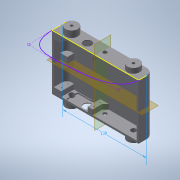
# Autodesk Inventor part: base-v2
Saved by Autodesk Inventor 2020 (Build 240168000, 168)
## iProperties
Created: 2020-08-23
Part Number: base-v2
Material: Ogólny
Document SubType Name: Modeling
Designer: blep
Density: 1 g/cm^3
Appearance: Domyślna
Author: blep
Autodesk Inventor part; units mm, degrees
ref_plane "YZ Plane" through (0, 0, 0) normal (1, 0, 0) x (0, 1, 0)
ref_plane "XZ Plane" through (0, 0, 0) normal (0, 1, 0) x (-1, 0, 0)
ref_plane "XY Plane" through (0, 0, 0) normal (0, 0, 1) x (1, 0, 0)
sketch "Szkic1" plane through (0, 0, 0) normal (0, 0, 1) x (1, 0, 0)
  line L0 (0, 0) -> (135, 0)
  line L1 (135, 0) -> (135, -86)
  line L2 (135, -86) -> (0, -86)
  line L3 (0, -86) -> (0, 0)
  line L4 (3, -3) -> (132, -3)
  line L5 (132, -3) -> (132, -83)
  line L6 (132, -83) -> (3, -83)
  line L7 (3, -83) -> (3, -3)
  dimension "d0" = 86
  dimension "d1" = 135
  dimension "d2" = 3
  constraints: 16 end point, 4 parallel, 2 perpendicular, 1 horizontal, 3 other
  measures "d0" distance of L0.end L1.end
  measures "d1" distance of L1.end L2.end
  measures "d2" distance between parallel lines of L3 L7
extrude "Wyciągnięcie proste1" add sketch "Szkic1" against normal blind 3 contours L0 L1 L2 L3 | L4 L5 L6 L7
extrude "Wyciągnięcie proste2" add sketch "Szkic1" along normal blind 20
sketch "Szkic2" plane through (0, 0, -3) normal (0, 1, 0) x (1, 0, 0)
  line L0 (135, 0) -> (135, -23) projected
  line L1 (0, 0) -> (135, 0) projected
  line L2 (0, 0) -> (0, -23) projected
  line L3 (135, -23) -> (0, -23) projected
  line L4 (115.75, -11.5) -> (19.25, -11.5)
  line L5 (135, -23) -> (115.75, -11.5) construction
  line L6 (0, 0) -> (135, 0) construction
  line L7 (115.75, -11.5) -> (135, 0) construction
  line L8 (135, -23) -> (0, -23) construction
  line L9 (19.25, -11.5) -> (0, -23) construction
  point P0 (0, -3)
  dimension "d7" = 96.5
  constraints: 8 end point, 2 equal length, 1 horizontal
  measures "d7" distance of L4.start L4.end
hole "Otwór1" at (19.25, 0, 8.5) at (115.75, 0, 8.5) direction (0, -1, 0) diameter 4.25 end through all
sketch "Szkic3" plane through (0, 0, -3) normal (0, 1, 0) x (1, 0, 0)
  circle A0 centre (19.25, -11.5) radius 2.125 projected
  circle A1 centre (19.25, -11.5) radius 10 projected
  circle A2 centre (19.25, -11.5) radius 9.5
  circle A3 centre (115.75, -11.5) radius 2.125 projected
  circle A4 centre (115.75, -11.5) radius 2.125 projected
  circle A5 centre (115.75, -11.5) radius 9.5
  point P0 (0, -3)
  dimension "d15" = 0.5
  constraints: 2 centre point, 1 coincident, 1 equal radius
  measures "d15" radial gap between concentric circles of A1 A2
extrude "Wyciągnięcie proste3" add sketch "Szkic3" along normal blind 10 contours A2
extrude "Wyciągnięcie proste4" add sketch "Szkic3" along normal blind 7.6 contours A5
ref_plane "Płaszczyzna konstrukcyjna1" through (0, -43, -3) normal (0, 1, 0) x (1, 0, 0)
mirror "Odbij1" about plane through (0, -43, -3) normal (0, 1, 0) of "Wyciągnięcie proste3", "Wyciągnięcie proste4"
ref_plane "Płaszczyzna konstrukcyjna2" through (0, -43, -3) normal (0, 1, 0) x (1, 0, 0)
sketch "Szkic4" plane through (3, -83, 0) normal (0, 1, 0) x (1, 0, 0)
  circle A0 centre (16.25, -8.5) radius 2.125 projected
  circle A1 centre (112.75, -8.5) radius 2.125 projected
  circle A2 centre (112.75, -8.5) radius 4
  circle A3 centre (16.25, -8.5) radius 4
  point P0 (-3, 0)
  dimension "d20" = 8
  dimension "d21" = 8
  constraints: 2 centre point, 2 coincident
  measures "d20" diameter of A2
  measures "d21" diameter of A3
extrude "Wyciągnięcie proste5" cut sketch "Szkic4" against normal blind 10 contours A0 | A3
extrude "Wyciągnięcie proste6" cut sketch "Szkic4" against normal blind 7.6 contours A1 | A2
mirror "Odbij2" about plane through (0, -43, -3) normal (0, 1, 0) of "Wyciągnięcie proste5", "Wyciągnięcie proste6"
sketch "Szkic5" plane through (3, -83, 0) normal (0, 1, 0) x (1, 0, 0)
  arc A0 (12, -18.8) -> (12.7, -19.5) centre (12.7, -18.8) ccw projected
  line L0 (12, -18.8) -> (12, -1) projected
  arc A1 (12.7, -0.3) -> (12, -1) centre (12.7, -1) ccw projected
  line L1 (12.7, -0.3) -> (42.3, -0.3) projected
  arc A2 (42.3, -0.3) -> (38.7014, -1) centre (42.3, -9.9) ccw projected
  line L2 (38.7014, -1) -> (19.4014, -1) projected
  arc A3 (19.4014, -1) -> (18.4014, -2) centre (19.4014, -2) ccw projected
  line L3 (18.4014, -2) -> (18.4014, -4.6756) projected
  arc A4 (18.4014, -4.6756) -> (18.4014, -14.0756) centre (22.3218, -9.3756) ccw projected
  line L4 (18.4014, -14.0756) -> (18.4014, -17.8) projected
  arc A5 (18.4014, -17.8) -> (19.4014, -18.8) centre (19.4014, -17.8) ccw projected
  line L5 (19.4014, -18.8) -> (38.7014, -18.8) projected
  arc A6 (38.7014, -18.8) -> (42.3, -19.5) centre (42.3, -9.9) ccw projected
  line L6 (42.3, -19.5) -> (12.7, -19.5) projected
  arc A7 (51.3, -19.5) -> (52, -18.8) centre (51.3, -18.8) ccw projected
  line L7 (51.3, -19.5) -> (42.3, -19.5) projected
  arc A8 (42.3, -19.5) -> (42.3, -0.3) centre (42.3, -9.9) ccw projected
  line L8 (42.3, -0.3) -> (51.3, -0.3) projected
  arc A9 (52, -1) -> (51.3, -0.3) centre (51.3, -1) ccw projected
  line L9 (52, -1) -> (52, -18.8) projected
  arc A10 (42.3, -19.75) -> (42.3, -0.05) centre (42.3, -9.9) ccw
  arc A11 (38.6531, -19.05) -> (42.3, -19.75) centre (42.3, -9.9) ccw
  line L10 (38.6531, -19.05) -> (19.4014, -19.05)
  arc A12 (18.1514, -17.8) -> (19.4014, -19.05) centre (19.4014, -17.8) ccw
  line L11 (18.1514, -17.8) -> (18.1514, -14.1912)
  arc A13 (18.1514, -4.56) -> (18.1514, -14.1912) centre (22.3218, -9.3756) ccw
  line L12 (18.1514, -4.56) -> (18.1514, -2)
  arc A14 (19.4014, -0.75) -> (18.1514, -2) centre (19.4014, -2) ccw
  line L13 (19.4014, -0.75) -> (38.6531, -0.75)
  arc A15 (42.3, -0.05) -> (38.6531, -0.75) centre (42.3, -9.9) ccw
  point P0 (-3, 0)
  point P1 (52, -11.6125)
  point P2 (52, -8.1875)
  point P3 (44.5051, -0.3)
  point P4 (40.0949, -0.3)
  dimension "d0" = 86
  dimension "d1" = 135
  dimension "d2" = 3
  dimension "d26" = 0.25
  dimension "d27" = 0.25
  constraints: 12 point on circle, 8 end point, 6 centre point, 8 other
  measures "d26" radial gap between concentric circles of A8 A10
  measures "d27" distance between parallel lines of L5 L10
extrude "Wyciągnięcie proste7" cut sketch "Szkic5" against normal blind 2 contours A11 L10 A12 L11 A13 L12 A14 L13 A15 L1 A2 L2 A3 L3 A4 L4 A5 L5 A6 L6 | L6 L7 A10 A11 | A8 L8 A10 L9 L7 | A6 L5 A5 L4 A4 L3 A3 L2 A2 A8
sketch "Szkic6" plane through (0, -86, -3) normal (0, -1, 0) x (1, 0, 0)
  circle A0 centre (45.3, 12.9) radius 6.4 projected
  point P0 (0, 3)
extrude "Wyciągnięcie proste8" cut sketch "Szkic6" against normal up to surface (3 mm away)
mirror "Odbij3" about plane through (0, -43, -3) normal (0, 1, 0) of "Wyciągnięcie proste7", "Wyciągnięcie proste8"
sketch "Szkic7" plane through (0, 0, 0) normal (0, 0, 1) x (1, 0, 0)
  line L0 (14.3963, -13.7) -> (14.3963, -34.2) projected
  line L1 (54.9963, -34.2) -> (54.9963, -13.7) projected
  line L2 (54.9963, -72.3) -> (54.9963, -51.8) projected
  line L3 (14.3963, -51.8) -> (14.3963, -72.3) projected
  line L4 (8.7, -10.9) -> (14.7, -10.9) projected
  line L5 (14.7, -5.2) -> (14.7, -10.9) projected
  line L6 (55.3, -10.9) -> (55.3, -5.2) projected
  line L7 (61.3, -10.9) -> (55.3, -10.9) projected
  line L8 (55.3, -13.7) -> (61.3, -13.7) projected
  line L9 (14.7, -13.7) -> (8.7, -13.7) projected
  line L10 (55.3, -13.7) -> (54.3, -13.7) projected
  line L11 (14.3963, -13.7) -> (15.3963, -13.7) projected
  line L12 (8.7, -72.3) -> (14.7, -72.3) projected
  line L13 (15.3963, -72.3) -> (14.3963, -72.3) projected
  line L14 (61.3, -72.3) -> (55.3, -72.3) projected
  line L15 (54.3, -72.3) -> (55.3, -72.3) projected
  line L16 (14.7, -75.1) -> (8.7, -75.1) projected
  line L17 (14.7, -75.1) -> (14.7, -80.8) projected
  line L18 (55.3, -75.1) -> (61.3, -75.1) projected
  line L19 (55.3, -80.8) -> (55.3, -75.1) projected
  line L20 (3, -3) -> (14.45, -3)
  line L21 (14.45, -3) -> (14.45, -10.65)
  line L22 (14.45, -10.65) -> (3, -10.65)
  line L23 (3, -10.65) -> (3, -3)
  line L24 (55.55, -3) -> (63.55, -3)
  line L25 (63.55, -3) -> (63.55, -10.65)
  line L26 (63.55, -10.65) -> (55.55, -10.65)
  line L27 (55.55, -10.65) -> (55.55, -3)
  line L28 (3, -75.35) -> (14.45, -75.35)
  line L29 (14.45, -75.35) -> (14.45, -83)
  line L30 (14.45, -83) -> (3, -83)
  line L31 (3, -83) -> (3, -75.35)
  line L32 (55.55, -75.35) -> (63.55, -75.35)
  line L33 (63.55, -75.35) -> (63.55, -83)
  line L34 (63.55, -83) -> (55.55, -83)
  line L35 (55.55, -83) -> (55.55, -75.35)
  line L36 (132, -83) -> (3, -83) projected
  line L37 (3, -3) -> (3, -83) projected
  line L38 (132, -3) -> (3, -3) projected
  line L39 (3, -34.2) -> (14.1463, -34.2)
  line L40 (14.1463, -34.2) -> (14.1463, -51.8)
  line L41 (14.1463, -51.8) -> (3, -51.8)
  line L42 (3, -51.8) -> (3, -34.2)
  line L43 (14.1463, -34.2) -> (14.3963, -34.2) construction
  line L44 (14.1463, -51.8) -> (14.3963, -51.8) construction
  line L45 (3, -83) -> (3, -3) construction
  line L46 (55.2463, -34.2) -> (63.55, -34.2)
  line L47 (63.55, -34.2) -> (63.55, -51.8)
  line L48 (63.55, -51.8) -> (55.2463, -51.8)
  line L49 (55.2463, -51.8) -> (55.2463, -34.2)
  point P0 (0, 0)
  point P1 (3, -51.8)
  dimension "d32" = 0.25
  dimension "d33" = 0.25
  dimension "d34" = 0.25
  dimension "d35" = 0.25
  dimension "d36" = 0.25
  dimension "d37" = 0.25
  dimension "d38" = 8
  dimension "d39" = 0.25
  dimension "d40" = 0.25
  constraints: 52 end point, 12 parallel, 10 collinear, 8 horizontal, 6 perpendicular, 3 point on line
  measures "d32" distance between parallel lines of L16 L28
  measures "d33" distance between parallel lines of L17 L29
  measures "d34" distance between parallel lines of L19 L35
  measures "d35" distance between parallel lines of L18 L32
  measures "d36" distance between parallel lines of L4 L22
  measures "d37" distance between parallel lines of L7 L26
  measures "d38" distance between parallel lines of L33 L35
  measures "d39" distance between parallel lines of L0 L40
  measures "d40" distance between parallel lines of L1 L49
extrude "Wyciągnięcie proste9" add sketch "Szkic7" along normal blind 20 contours L20 L21 L22 L23 | L24 L25 L26 L27 | L28 L29 L30 L31 | L32 L33 L34 L35
extrude "Wyciągnięcie proste10" add sketch "Szkic7" along normal blind 10 contours L39 L40 L41 L37
chamfer "Faza1" distance 5 angle 45 2 edges at (63.55, -6.825, 0) (63.55, -79.175, 0)
sketch "Szkic9" plane through (55.55, -75.35, 20) normal (0, 1, 0) x (1, 0, 0)
  arc A0 (-47.2504, 3.85) -> (-47.2504, 6.35) centre (-45.44, 5.1) ccw projected
  arc A1 (-47.2504, 13.85) -> (-47.2504, 16.35) centre (-45.44, 15.1) ccw projected
  arc A2 (6.1504, 6.35) -> (6.1504, 3.85) centre (4.34, 5.1) ccw projected
  arc A3 (6.1504, 16.35) -> (6.1504, 13.85) centre (4.34, 15.1) ccw projected
  point P0 (-55.55, 20)
hole "Otwór2" at (59.89, -75.35, 4.9) at (59.89, -75.35, 14.9) at (10.11, -75.35, 14.9) at (10.11, -75.35, 4.9) direction (0, -1, 0) diameter 1.5 depth 7.5
mirror "Odbij4" about plane through (0, -43, -3) normal (0, 1, 0) of "Otwór2"
sketch "Szkic10" plane through (0, 0, -3) normal (0, 1, 0) x (1, 0, 0)
  circle A0 centre (115.75, -11.5) radius 9.5 projected
  arc A1 (135, -10) -> (125, 0) centre (125, -10) ccw
  arc A2 (132, -10) -> (125, -3) centre (125, -10) ccw
  line L0 (132, -10) -> (135, -10)
  line L1 (132, -3) -> (132, -23) projected
  line L2 (125, -3) -> (125, 0)
  line L3 (0, 0) -> (135, 0) projected
  line L4 (135, 0) -> (135, -23) projected
  point P0 (0, -3)
  dimension "d55" = 10
  dimension "d56" = 3
  dimension "d57" = 10
  dimension "d58" = 10
  constraints: 4 end point, 4 point on circle, 2 centre point, 2 perpendicular, 2 tangent
  measures "d55" radius of A1
  measures "d56" radial gap between concentric circles of A1 A2
  measures "d57" distance between parallel lines of L3 L0
  measures "d58" distance between parallel lines of L4 L2
extrude "Wyciągnięcie proste11" cut sketch "Szkic10" against normal through all contours A1 L3 L4
extrude "Wyciągnięcie proste12" add sketch "Szkic10" against normal up to surface (86 mm away) contours L0 A2 L2 A1
sketch "Szkic11" plane through (63.55, -83, 20) normal (0, 1, 0) x (1, 0, 0)
  circle A0 centre (52.2, 11.5) radius 4 projected
  arc A1 (-43.7975, 7.5317) -> (-42.6968, 15.1647) centre (-44.3, 11.5) ccw projected
  line L0 (52.2, 11.5) -> (-44.3, 11.5) construction
  point P0 (-63.55, 20)
  point P1 (7.7, 11.5)
  dimension "d63" = 52
  constraints: 2 end point, 1 horizontal, 1 point on line
  measures "d63" distance of point (7.7, 11.5) L0.end
hole "Otwór3" at (71.25, -83, 8.5) direction (0, -1, 0) diameter 6 end through all
mirror "Odbij5" about plane through (0, -43, -3) normal (0, 1, 0) of "Otwór3"
ref_plane "Płaszczyzna konstrukcyjna3" through (67.5, -86, -3) normal (-1, 0, 0) x (0, 0, 1)
mirror "Odbij6" about plane through (67.5, -86, -3) normal (-1, 0, 0) of "Wyciągnięcie proste11", "Wyciągnięcie proste12"
sketch "Szkic12" plane through (0, 0, 20) normal (0, 1, 0) x (1, 0, 0)
  line L0 (135, 0) -> (0, 0) projected
  line L1 (135, 13) -> (135, 0) projected
  line L2 (0, 13) -> (0, 0) projected
  line L3 (135, 0) -> (132.4233, -28.9235) construction
  line L4 (132.4233, -28.9235) -> (75.3848, -36.0533) construction
  line L5 (75.3848, -36.0533) -> (37.2527, -38.8798) construction
  line L6 (37.2527, -38.8798) -> (1.4131, -37.5387) construction
  line L7 (1.4131, -37.5387) -> (0, 0) construction
  spline S0 degree 4 poles (135, 0) (132.4233, -28.9235) (75.3848, -36.0533) (37.2527, -38.8798) (1.4131, -37.5387) (0, 0) knots 1 1 1 1 1 2 3 3 3 3 3
  point P0 (0, 20)
  constraints: 3 other
equation "\"d33\" = d32"
equation "\"d34\" = d32"
equation "\"d35\" = d32"
equation "\"d36\" = d32"
equation "\"d37\" = d32"
equation "\"d40\" = d39"
